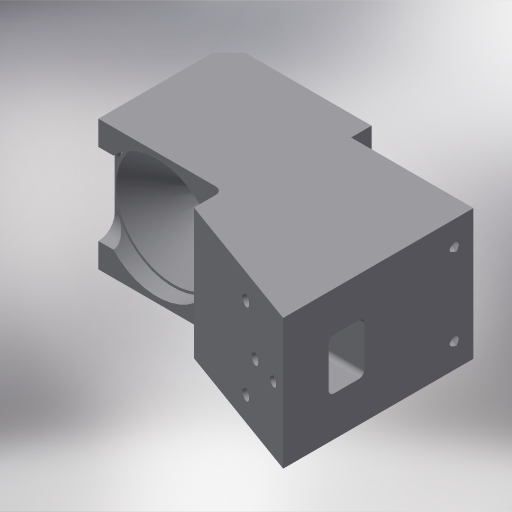
# Autodesk Inventor part: OdorBase_SideVacuumPort
Saved by Autodesk Inventor 2023 (Build 270158000, 158)
## iProperties
Created: 2008-10-04
Part Number: OdorBase_SideVacuumPort
Document SubType Name: Modeling
Designer: rinbergd
Density: 1 g/cm^3
Material: Generic
Appearance: Default
Author: osbornej
Autodesk Inventor part; units mm, degrees
ref_plane "YZ Plane" through (0, 0, 0) normal (1, 0, 0) x (0, 1, 0)
sketch "Sketch1" plane through (0, 0, 0) normal (0, 0, 1) x (1, 0, 0)
  line L0 (0, 24.892) -> (0, -24.892) projected
  line L1 (-25.6032, 0) -> (39.8272, 0) projected
  line L2 (30.48, -17.78) -> (-16.256, -17.78)
  line L3 (-16.256, -17.78) -> (-16.256, 17.78)
  line L4 (-16.256, 17.78) -> (30.48, 17.78)
  line L5 (30.48, 17.78) -> (30.48, -17.78)
  dimension "d0" = 30.48
  dimension "d1" = 16.256
  dimension "d2" = 17.78
  dimension "d3" = 35.56
  constraints: 8 end point, 2 parallel, 1 horizontal, 1 perpendicular
  measures "d0" distance between parallel lines of L5 L0
  measures "d1" distance between parallel lines of L3 L0
  measures "d2" distance between parallel lines of L1 L4
  measures "d3" distance of L2.end L3.end
extrude "Extrusion1" add sketch "Sketch1" along normal blind 45.72
sketch "Sketch2" plane through (-16.256, -17.78, 0) normal (0, -1, 0) x (1, 0, 0)
  line L0 (46.736, 45.72) -> (0, 45.72) projected
  line L1 (0, 0) -> (0, 45.72) projected
  line L2 (46.736, 0) -> (0, 0) projected
  line L3 (16.256, 54.864) -> (16.256, -9.144) projected
  line L4 (16.256, 45.72) -> (16.256, 20.32)
  line L5 (16.256, 20.32) -> (4.064, 20.32)
  line L6 (4.064, 20.32) -> (4.064, 23.368)
  arc A0 (4.064, 23.368) -> (0, 23.368) centre (2.032, 23.368) ccw
  line L7 (0, 23.368) -> (0, 45.72)
  line L8 (0, 45.72) -> (16.256, 45.72)
  line L9 (0, 2.54) -> (2.54, 0)
  line L10 (2.54, 0) -> (0, 0)
  line L11 (0, 0) -> (0, 2.54)
  dimension "d6" = 25.4
  dimension "d7" = 2.032
  dimension "d8" = 2.032
  dimension "d9" = 3.048
  dimension "d10" = 2.54
  dimension "d11" = 2.54
  dimension "d12" = 4.064
  constraints: 16 end point, 5 perpendicular, 5 point on line, 2 point on circle, 1 centre point, 1 collinear
  measures "d6" distance of L4.start L4.end
  measures "d7" radius of A0
  measures "d8" distance from line of L1 A0.centre
  measures "d9" distance from line of L5 A0.centre
  measures "d10" distance of L1.start L9.start
  measures "d11" distance of L9.end L1.start
  measures "d12" distance between parallel lines of L6 L7
extrude "Extrusion2" cut sketch "Sketch2" against normal through all contours L3 L5 L6 A0 L1 L0 | L9 L2 L1
sketch "Sketch3" plane through (-16.256, -17.78, 23.368) normal (-1, 0, 0) x (0, 0, 1)
  line L0 (-20.828, 35.56) -> (0, 35.56) projected
  line L1 (-20.828, 0) -> (0, 0) projected
  line L2 (-32.512, 17.78) -> (31.496, 17.78) projected
  line L3 (2.032, 35.56) -> (2.032, 0) projected
  line L4 (2.032, 35.56) -> (0, 35.56) projected
  line L5 (-23.368, 35.56) -> (-20.828, 35.56) projected
  line L6 (-20.828, 0) -> (-23.368, 0) projected
  line L7 (0, 0) -> (2.032, 0) projected
  line L8 (2.032, 0) -> (-23.368, 0)
  line L9 (-23.368, 0) -> (-23.368, 5.08)
  line L10 (-23.368, 5.08) -> (-3.048, 5.08)
  line L11 (-3.048, 5.08) -> (-3.048, 6.35)
  line L12 (-3.048, 6.35) -> (2.032, 6.35)
  line L13 (2.032, 6.35) -> (2.032, 0)
  line L14 (-20.828, 35.56) -> (0, 35.56)
  line L15 (-20.828, 35.56) -> (-23.368, 35.56)
  line L16 (0, 35.56) -> (2.032, 35.56)
  line L17 (2.032, 35.56) -> (-23.368, 35.56)
  line L18 (-23.368, 35.56) -> (-23.368, 30.48)
  line L19 (-23.368, 30.48) -> (-3.048, 30.48)
  line L20 (-3.048, 30.48) -> (-3.048, 29.21)
  line L21 (-3.048, 29.21) -> (2.032, 29.21)
  line L22 (2.032, 29.21) -> (2.032, 35.56)
  dimension "d15" = 6.35
  dimension "d16" = 5.08
  dimension "d17" = 5.08
  constraints: 30 end point, 4 perpendicular, 4 symmetric about line, 1 collinear, 1 parallel, 1 point on line
  measures "d15" distance of L12.end L3.end
  measures "d16" distance of L6.end L9.end
  measures "d17" distance between parallel lines of L11 L3
extrude "Extrusion3" cut sketch "Sketch3" against normal up to surface (16.256 mm away)
sketch "Sketch4" plane through (-16.256, -12.7, 2.54) normal (-1, 0, 0) x (0, 0, 1)
  line L0 (-11.684, 12.7) -> (52.324, 12.7) projected
  line L1 (22.86, 24.13) -> (22.86, 1.27) projected
  line L2 (22.86, 12.7) -> (22.86, 6.35)
  line L3 (17.78, 6.35) -> (22.86, 6.35)
  line L4 (15.24, 8.89) -> (15.24, 12.7)
  line L5 (15.24, 12.7) -> (22.86, 12.7)
  arc A0 (15.24, 8.89) -> (17.78, 6.35) centre (17.78, 8.89) ccw
  line L6 (22.86, 12.7) -> (22.86, 19.05)
  line L7 (17.78, 19.05) -> (22.86, 19.05)
  line L8 (15.24, 16.51) -> (15.24, 12.7)
  arc A1 (17.78, 19.05) -> (15.24, 16.51) centre (17.78, 16.51) ccw
  dimension "d20" = 2.54
  dimension "d21" = 6.35
  dimension "d22" = 7.62
  constraints: 14 end point, 4 point on circle, 4 symmetric about line, 3 perpendicular, 2 centre point, 2 point on line, 2 tangent, 1 midpoint, 1 other
  measures "d20" radius of A0
  measures "d21" distance of L2.start L2.end
  measures "d22" distance of L4.end L2.start
extrude "Extrusion4" cut sketch "Sketch4" against normal blind 7.874
sketch "Sketch11" plane through (0, -17.78, 0) normal (-1, 0, 0) x (0, 0, 1)
  line L0 (20.32, 5.08) -> (20.32, 30.48) projected
  line L1 (45.72, 35.56) -> (45.72, 0) projected
  line L2 (-9.144, 17.78) -> (54.864, 17.78) projected
  line L3 (20.32, 25.4) -> (20.32, 10.16) projected
  point P0 (20.32, 24.3791)
  point P1 (20.32, 11.1809)
  point P2 (43.18, 16.51)
  point P3 (43.18, 19.05)
  point P4 (23.368, 17.78)
  point P5 (22.733, 17.78)
  dimension "d73" = 1.27
  dimension "d74" = 1.27
  dimension "d75" = 2.54
  dimension "d76" = 2.54
  dimension "d78" = 0.635
  dimension "d476" = 2.413
  constraints: 2 point on line
  measures "d73" distance from line of point (43.18, 16.51) L2
  measures "d74" distance from line of point (43.18, 19.05) L2
  measures "d75" distance from line of point (43.18, 16.51) L1
  measures "d76" distance from line of point (43.18, 19.05) L1
  measures "d78" distance of point (22.733, 17.78) point (23.368, 17.78)
  measures "d476" distance from line of L0 point (22.733, 17.78)
hole "Hole3" at (0, 0, 22.733) direction (1, 0, 0) diameter 1.524 end through all
sketch "Sketch21" plane through (0, 0, 0) normal (0, 1, 0) x (-1, 0, 0)
  line L0 (0, -4.064) -> (0, 24.384) projected
  line L1 (13.716, 0) -> (0, 0) projected
  line L2 (16.256, 20.32) -> (16.256, 2.54) projected
  line L3 (4.3942, 0) -> (7.1374, 0)
  line L4 (4.3942, 0) -> (4.3942, 6.35)
  line L5 (4.3942, 6.35) -> (5.5499, 6.35)
  line L6 (5.5499, 6.35) -> (5.5499, 10.4775)
  line L7 (0, 20.32) -> (16.256, 20.32) projected
  line L8 (7.1374, 0) -> (7.1374, 20.32)
  line L9 (5.5499, 10.4775) -> (-1.7526, 17.78)
  line L10 (-1.7526, 17.78) -> (-1.7526, 20.32)
  line L11 (-1.7526, 20.32) -> (7.1374, 20.32)
  line L12 (-1.7526, 17.78) -> (-2.1495, 17.78)
  line L13 (-2.1495, 17.78) -> (-2.1495, 20.32)
  line L14 (-2.1495, 20.32) -> (-1.7526, 20.32)
  line L15 (-1.7526, 20.32) -> (-1.7526, 17.78)
  line L16 (5.5499, 8.4138) -> (7.1374, 8.4138)
  dimension "d159" = 7.1374
  dimension "d160" = 8.89
  dimension "d162" = 45
  dimension "d163" = 1.5875
  dimension "d292" = 0.3969
  dimension "d322" = 2.54
  constraints: 26 end point, 5 perpendicular, 5 point on line, 2 parallel, 1 collinear, 1 horizontal, 1 midpoint
  measures "d159" distance between parallel lines of L8 L0
  measures "d160" distance between parallel lines of L8 L10
  measures "d162" angle of L8 L9
  measures "d163" distance between parallel lines of L8 L6
  measures "d292" distance between parallel lines of L10 L13
  measures "d322" distance of L12.end L13.end
revolve "Revolution5" cut sketch "Sketch21" angle 360 about axis through (-7.1374, 0, 0) along (0, 0, 1) contours L9 L10 L11 L0 | L0 L7 L8 L16 L6 L9 | L4 L5 L6 L16 L8 L1 | L12 L13 L14 L10
sketch "Sketch23" plane through (0, 0, 0) normal (0, 0, -1) x (-1, 0, 0)
  line L0 (13.716, 12.7) -> (0, 12.7) projected
  line L1 (0, 17.78) -> (-30.48, 17.78) projected
  line L2 (-39.8272, 0) -> (25.6032, 0) projected
  line L3 (16.256, 12.7) -> (16.256, -12.7) projected
  line L4 (0, -12.7) -> (13.716, -12.7) projected
  line L5 (-30.48, -17.78) -> (0, -17.78) projected
  line L6 (8.382, -12.7) -> (8.382, -11.43)
  line L7 (-30.48, 17.78) -> (-30.48, -17.78) projected
  line L8 (8.382, -11.43) -> (-30.48, -11.43)
  line L9 (-30.48, -11.43) -> (-30.48, -17.78)
  line L10 (-30.48, -17.78) -> (8.382, -17.78)
  line L11 (8.382, -17.78) -> (8.382, -12.7)
  dimension "d193" = 7.874
  dimension "d231" = 6.35
  constraints: 10 end point, 3 perpendicular, 3 point on line
  measures "d193" distance between parallel lines of L3 L6
  measures "d231" distance between parallel lines of L8 L5
extrude "Extrusion12" cut sketch "Sketch23" against normal blind 27.94
mirror "Mirror5" about plane through (0, 0, 0) normal (0, 1, 0) of "Extrusion12"
sketch "Sketch32" plane through (0, 17.78, 45.72) normal (0, 1, 0) x (1, 0, 0)
  line L0 (30.48, 17.78) -> (0, 17.78) projected
  line L1 (0, 17.78) -> (0, 0) projected
  line L2 (0, 0) -> (30.48, 0) projected
  line L3 (30.48, 17.78) -> (30.48, 0) projected
extrude "Extrusion16" cut sketch "Sketch32" against normal up to surface (6.35 mm away)
sketch "Sketch33" plane through (0, -17.78, 45.72) normal (0, -1, 0) x (1, 0, 0)
  circle A0 centre (3.1266, -12.4245) radius 0.7366 projected
  line L0 (0, -17.78) -> (30.48, -17.78) projected
  line L1 (30.48, -17.78) -> (30.48, 0) projected
  line L2 (30.48, 0) -> (0, 0) projected
  line L3 (0, 0) -> (0, -17.78) projected
extrude "Extrusion17" cut sketch "Sketch33" against normal up to surface (6.35 mm away)
sketch "Sketch34" plane through (0, 11.43, 45.72) normal (0, 1, 0) x (1, 0, 0)
  line L0 (0, 0) -> (0, 25.4) projected
  line L1 (30.48, 0) -> (0, 0) projected
  line L2 (30.48, 45.72) -> (30.48, 0) projected
  line L3 (26.9647, 12.195) -> (4.5883, 20.3394) projected
  line L4 (26.9647, 12.195) -> (30.48, 10.9156)
  line L5 (4.5883, 20.3394) -> (0, 22.0094)
  point P0 (0, 24.13)
  constraints: 4 end point, 2 collinear, 2 point on line
extrude "Extrusion18" cut sketch "Sketch34" along normal through all both and the other way through all
sketch "Sketch35" plane through (-8.382, -11.43, 0) normal (0, -1, 0) x (1, 0, 0)
  line L0 (38.862, 34.8044) -> (8.382, 23.7106) projected
  line L1 (8.382, 20.32) -> (8.382, 23.7106) projected
  line L2 (38.862, 34.8044) -> (38.862, 0) projected
  line L3 (8.382, 20.32) -> (10.4457, 20.32)
  line L4 (11.557, 21.4312) -> (11.557, 24.8662)
  arc A0 (10.4457, 20.32) -> (11.557, 21.4312) centre (10.4457, 21.4312) ccw
  dimension "d284" = 1.1113
  dimension "d285" = 3.175
  constraints: 4 end point, 2 perpendicular, 2 point on circle, 2 point on line, 2 tangent, 1 centre point
  measures "d284" radius of A0
  measures "d285" distance between parallel lines of L4 L1
extrude "Extrusion19" cut sketch "Sketch35" against normal through all
sketch "Sketch38" plane through (0, 0, 0) normal (0, 0, -1) x (-1, 0, 0)
  line L0 (8.382, 11.43) -> (17.907, 11.43)
  line L1 (17.907, 11.43) -> (17.907, 14.605)
  line L2 (17.907, 14.605) -> (8.382, 14.605)
  line L3 (8.382, -11.43) -> (17.907, -11.43)
  line L4 (17.907, -11.43) -> (17.907, -14.605)
  line L5 (17.907, -14.605) -> (8.382, -14.605)
  line L6 (13.716, 12.7) -> (8.382, 12.7) projected
  line L7 (8.382, 11.43) -> (8.382, 14.605)
  line L8 (8.382, -11.43) -> (8.382, -14.605)
  dimension "d293" = 3.175
  dimension "d294" = 3.175
  dimension "d295" = 9.525
  constraints: 16 end point, 3 equal length, 3 perpendicular, 2 horizontal, 1 collinear
  measures "d293" distance of L0.end L1.end
  measures "d294" distance of L3.end L4.end
  measures "d295" distance of L1.end L2.end
extrude "Extrusion22" cut sketch "Sketch38" against normal through all
sketch "Sketch39" plane through (-16.256, -11.43, 2.54) normal (0, -1, 0) x (1, 0, 0)
  line L0 (4.064, 17.78) -> (18.3197, 17.78) projected
  line L1 (4.064, 20.828) -> (4.064, 17.78) projected
  arc A0 (4.064, 20.828) -> (0, 20.828) centre (2.032, 20.828) ccw projected
  line L2 (0, 0) -> (0, 20.828) projected
  line L3 (2.54, -2.54) -> (0, 0) projected
  line L4 (46.736, -2.54) -> (2.54, -2.54) projected
  line L5 (46.736, 32.2644) -> (46.736, -2.54) projected
  line L6 (46.736, 32.2644) -> (19.431, 22.3262) projected
  line L7 (19.431, 22.3262) -> (19.431, 18.8912) projected
  arc A1 (18.3197, 17.78) -> (19.431, 18.8912) centre (18.3197, 18.8912) ccw projected
  line L8 (4.4328, 17.78) -> (0, 17.78)
  constraints: 2 end point, 2 point on line, 1 perpendicular
extrude "Extrusion23" cut sketch "Sketch39" against normal through all contours L8 L2 A0 L1
sketch "Sketch45" plane through (-16.256, -11.43, 2.54) normal (0, -1, 0) x (1, 0, 0)
  line L0 (0, 17.78) -> (18.3197, 17.78) projected
  line L1 (0, 0) -> (0, 17.78) projected
  line L2 (2.54, -2.54) -> (0, 0) projected
  line L3 (46.736, -2.54) -> (2.54, -2.54) projected
  line L4 (46.736, 32.2644) -> (46.736, -2.54) projected
  line L5 (46.736, 32.2644) -> (19.431, 22.3262) projected
  line L6 (19.431, 22.3262) -> (19.431, 18.8912) projected
  arc A0 (18.3197, 17.78) -> (19.431, 18.8912) centre (18.3197, 18.8912) ccw projected
  circle A1 centre (2.3813, 7.62) radius 1.1906 projected
extrude "Extrusion29" cut sketch "Sketch45" against normal blind 1.27 contours L0 A0 L6 L5 L4 L3 L2 L1 | A1
sketch "Sketch46" plane through (-16.256, 11.43, 20.32) normal (0, 1, 0) x (1, 0, 0)
  line L0 (0, 0) -> (18.3197, 0) projected
  arc A0 (19.431, -1.1112) -> (18.3197, 0) centre (18.3197, -1.1112) ccw projected
  line L1 (19.431, -1.1112) -> (19.431, -4.5462) projected
  line L2 (19.431, -4.5462) -> (46.736, -14.4844) projected
  line L3 (46.736, 20.32) -> (46.736, -14.4844) projected
  line L4 (2.54, 20.32) -> (46.736, 20.32) projected
  line L5 (0, 17.78) -> (2.54, 20.32) projected
  line L6 (0, 0) -> (0, 17.78) projected
  circle A1 centre (2.3813, 10.16) radius 1.1906 projected
extrude "Extrusion30" cut sketch "Sketch46" against normal blind 1.27 contours L6 L5 L4 L3 L2 L1 A0 L0 | A1
sketch "Sketch47" plane through (-16.256, -10.16, 2.54) normal (0, -1, 0) x (1, 0, 0)
  line L0 (0, 0) -> (0, 17.78) projected
  line L1 (46.736, -2.54) -> (2.54, -2.54) projected
  line L2 (46.736, 32.2644) -> (46.736, -2.54) projected
  line L3 (19.431, 22.3262) -> (46.736, 32.2644) projected
  line L4 (0, 17.78) -> (18.3197, 17.78) projected
  line L5 (41.275, -2.54) -> (41.275, 30.2768)
  dimension "d327" = 41.275
  constraints: 2 end point, 2 point on line, 1 perpendicular
  measures "d327" distance between parallel lines of L5 L0
extrude "Extrusion31" cut sketch "Sketch47" against normal through all
sketch "Sketch49" plane through (0, 0, 0) normal (0, 0, -1) x (-1, 0, 0)
  circle A0 centre (-18.669, 0) radius 2.0574 projected
  line L0 (-5.969, -18.288) -> (-5.969, 13.462) projected
  line L1 (-31.369, -18.288) -> (-5.969, -18.288) projected
  line L2 (-31.369, -18.288) -> (-31.369, 13.462) projected
  line L3 (-31.369, 13.462) -> (-5.969, 13.462) projected
hole "Hole11" at (18.669, 0, 0) direction (0, 0, 1) diameter 3.6576 depth 7.9375 tip angle 118 clearance for "Flat Head Machine Screw (82)" size "#6" standard "Ansi Unified Screw Threads"
sketch "Sketch50" plane through (0, 0, 0) normal (0, 0, -1) x (-1, 0, 0)
  circle A0 centre (-18.669, 0) radius 1.8288 projected
  line L0 (13.716, 10.16) -> (-25.019, 10.16) projected
  line L1 (-25.019, 10.16) -> (-25.019, -10.16) projected
  line L2 (-25.019, -10.16) -> (13.716, -10.16) projected
  line L3 (-5.969, 10.16) -> (-5.969, -10.16)
  point P0 (-5.969, -10.16)
  point P1 (-5.969, 10.16)
  dimension "d340" = 19.05
  constraints: 2 end point, 2 point on line, 1 perpendicular
  measures "d340" distance between parallel lines of L3 L1
extrude "Extrusion33" cut sketch "Sketch50" against normal blind 3.175
sketch "Sketch51" plane through (25.019, -10.16, 32.8168) normal (1, 0, 0) x (0, 0, -1)
  circle A0 centre (10.0838, 10.16) radius 0.762 projected
  circle A1 centre (9.4488, 10.16) radius 0.508 projected
  line L0 (8.655, 8.5725) -> (11.0363, 8.5725)
  line L1 (11.0363, 8.5725) -> (11.0363, 11.7475)
  line L2 (11.0363, 11.7475) -> (8.655, 11.7475)
  line L3 (8.655, 11.7475) -> (8.655, 8.5725)
  circle A2 centre (8.655, 10.16) radius 1.5875
  circle A3 centre (11.0363, 10.16) radius 1.5875
  line L4 (-6.5634, 10.16) -> (39.3801, 10.16) projected
  line L5 (7.8613, 6.1913) -> (11.83, 6.1913)
  line L6 (12.6238, 6.985) -> (12.6238, 13.335)
  line L7 (11.83, 14.1288) -> (7.8613, 14.1288)
  line L8 (7.0675, 13.335) -> (7.0675, 6.985)
  arc A4 (7.0675, 7.7788) -> (8.655, 6.1913) centre (8.655, 7.7788) ccw
  arc A5 (12.6238, 13.335) -> (11.83, 14.1288) centre (11.83, 13.335) ccw
  arc A6 (11.83, 6.1913) -> (12.6238, 6.985) centre (11.83, 6.985) ccw
  arc A7 (7.8613, 14.1288) -> (7.0675, 13.335) centre (7.8613, 13.335) ccw
  arc A8 (7.0675, 6.985) -> (7.8613, 6.1913) centre (7.8613, 6.985) ccw
  dimension "d344" = 3.175
  dimension "d345" = 0
  dimension "d347" = 2.3813
  dimension "d352" = 0.9525
  dimension "d412" = 7.9375
  dimension "d413" = 3.9688
  dimension "d414" = 1.5875
  dimension "d415" = 0.7937
  constraints: 16 end point, 10 point on circle, 10 tangent, 5 centre point, 4 parallel, 3 equal radius, 2 horizontal, 2 midpoint, 2 perpendicular, 2 point on line, 2 vertical, 2 vertical alignment, 4 other
  measures "d344" distance between parallel lines of L2 L0
  measures "d345" distance from line of L4 point (11.036, 10.16)
  measures "d347" distance of L1.end L2.end
  measures "d352" distance from line of L1 A0.centre
  measures "d412" distance between parallel lines of L7 L5
  measures "d413" distance between parallel lines of L7 L4
  measures "d414" radius of A4
  measures "d415" radius of A5
extrude "Extrusion34" cut sketch "Sketch51" against normal blind 12.7
sketch "Sketch53" plane through (-16.256, -10.16, 2.54) normal (0, -1, 0) x (1, 0, 0)
  line L0 (0, 17.78) -> (18.3197, 17.78) projected
  line L1 (0, 17.78) -> (4.064, 17.78)
  line L2 (4.064, 17.78) -> (4.064, 20.828)
  line L3 (4.064, 20.828) -> (0, 20.828)
  line L4 (0, 20.828) -> (0, 17.78)
  circle A0 centre (2.032, 20.828) radius 2.032
  dimension "d353" = 4.064
  dimension "d354" = 3.048
  constraints: 8 end point, 2 parallel, 1 horizontal, 1 horizontal alignment, 1 midpoint, 1 perpendicular, 2 other
  measures "d353" distance of L2.end L3.end
  measures "d354" distance between parallel lines of L3 L0
extrude "Extrusion36" add sketch "Sketch53" against normal blind 3.81
sketch "Sketch54" plane through (-16.256, -10.16, 2.54) normal (0, -1, 0) x (1, 0, 0)
  line L0 (4.064, 17.78) -> (4.064, 20.828) projected
  arc A0 (4.064, 20.828) -> (0, 20.828) centre (2.032, 20.828) ccw projected
  line L1 (0, 20.828) -> (0, 0) projected
  line L2 (2.54, -2.54) -> (0, 0) projected
  line L3 (22.225, -2.54) -> (2.54, -2.54) projected
  line L4 (4.064, 17.78) -> (4.064, -2.54)
  constraints: 2 end point, 1 perpendicular, 1 point on line
extrude "Extrusion37" add sketch "Sketch54" along normal blind 3.175
sketch "Sketch55" plane through (-16.256, -13.335, 2.54) normal (0, -1, 0) x (1, 0, 0)
  arc A0 (4.064, 20.828) -> (0, 20.828) centre (2.032, 20.828) ccw projected
  point P0 (2.032, 20.828)
  constraints: 1 coincident
hole "Hole12" at (-14.224, -13.335, 23.368) direction (0, 1, 0) diameter 1.1906 depth 9.525 counterbore diameter 3.048 counterbore depth 5.334
sketch "Sketch56" plane through (2.0637, 1.2589, 20.32) normal (0, 0, 1) x (1, 0, 0)
  arc A0 (0, 0) -> (0, -2.5178) centre (-9.2011, -1.2589) ccw projected
  circle A1 centre (-9.2011, -1.2589) radius 9.2869
  point P0 (-14.2557, 6.5319)
  constraints: 1 centre point, 1 coincident, 1 concentric
extrude "Extrusion38" cut sketch "Sketch56" along normal blind 25.4
sketch "Sketch60" plane through (-16.256, -13.335, 2.54) normal (0, -1, 0) x (1, 0, 0)
  circle A0 centre (2.032, 20.828) radius 1.524 projected
  line L0 (4.064, 20.828) -> (4.064, -2.54) projected
  arc A1 (4.064, 20.828) -> (0, 20.828) centre (2.032, 20.828) ccw projected
  line L1 (0, 0) -> (0, 20.828) projected
  line L2 (0, 17.653) -> (4.064, 17.653)
  dimension "d378" = 3.175
  constraints: 2 end point, 2 point on line, 1 perpendicular
  measures "d378" distance from line of A0.centre L2
extrude "Extrusion41" cut sketch "Sketch60" against normal blind 1.27
sketch "Sketch62" plane through (-16.256, -13.335, 2.54) normal (0, -1, 0) x (1, 0, 0)
  line L0 (4.064, 11.303) -> (0, 11.303) projected
  line L1 (0, 0) -> (0, 17.653) projected
  line L2 (2.54, -2.54) -> (0, 0) projected
  line L3 (4.064, -2.54) -> (2.54, -2.54) projected
  line L4 (4.064, 17.653) -> (4.064, -2.54) projected
extrude "Extrusion43" cut sketch "Sketch62" against normal up to surface (3.175 mm away)
fillet "Fillet2" radius 0.4001 1 edges at (-14.224, -12.065, 20.193)
ref_plane "Work Plane10" through (-16.256, -14.605, 2.54) normal (0, -1, 0) x (1, 0, 0)
sketch "Sketch63" plane through (-16.256, -14.605, 2.54) normal (0, -1, 0) x (1, 0, 0)
  line L0 (0, 17.653) -> (4.064, 17.653) projected
  line L1 (0, 11.303) -> (0, 17.653) projected
  point P0 (2.032, 14.478)
  dimension "d387" = 3.175
  dimension "d388" = 2.032
  measures "d387" distance from line of point (2.032, 14.478) L0
  measures "d388" distance from line of point (2.032, 14.478) L1
hole "Hole13" at (-14.224, -14.605, 17.018) direction (0, 1, 0) diameter 2.159 depth 3.175 tip angle 118
mirror "Mirror8" about plane through (0, 0, 0) normal (0, 1, 0) of "Hole12", "Extrusion38", "Extrusion37", "Extrusion36", "Extrusion41", "Extrusion43", "Fillet2", "Hole13"
pattern_linear "Rectangular Pattern1" count 2 spacing 2.54 along (0, 1, 0) of "Hole3"
pattern_linear "Rectangular Pattern2" count 2 spacing 2.54 along (0, -1, 0) of "Hole3"
sketch "Sketch65" plane through (-16.256, -3.81, 17.78) normal (-1, 0, 0) x (0, 0, 1)
  line L0 (-3.937, 13.97) -> (8.3591, 13.97)
  line L1 (8.3591, 13.97) -> (8.3591, 19.1782)
  line L2 (8.3591, 19.1782) -> (-3.937, 19.1782)
  line L3 (-3.937, 19.1782) -> (-3.937, 13.97)
  line L4 (-4.3371, -6.35) -> (8.3591, -6.35)
  line L5 (8.3591, -6.35) -> (8.3591, -11.3681)
  line L6 (8.3591, -11.3681) -> (-4.3371, -11.3681)
  line L7 (-4.3371, -11.3681) -> (-4.3371, -6.35)
  line L8 (8.3591, 19.1782) -> (2.54, 19.1782)
  line L9 (2.54, 19.1782) -> (2.54, 10.16)
  line L10 (2.54, 10.16) -> (8.3591, 10.16)
  line L11 (8.3591, 10.16) -> (8.3591, 19.1782)
  line L12 (8.3591, -11.3681) -> (2.54, -11.3681)
  line L13 (2.54, -11.3681) -> (2.54, -2.54)
  line L14 (2.54, -2.54) -> (8.3591, -2.54)
  line L15 (8.3591, -2.54) -> (8.3591, -11.3681)
  constraints: 32 end point, 8 parallel, 4 horizontal, 4 perpendicular, 1 collinear
extrude "Extrusion44" cut sketch "Sketch65" against normal up to surface (4.064 mm away)
ref_plane "Work Plane6" through (-7.1374, 0, 10.4775) normal (0, -1, 0) x (0, 0, -1)
sketch "Sketch68" plane through (-16.256, -3.81, 17.78) normal (0, 0, 1) x (1, 0, 0)
  line L0 (0, 7.62) -> (0.6492, 7.62) projected
  line L1 (0, 0) -> (0, 7.62) projected
  line L2 (0, 0) -> (0.6492, 0) projected
  arc A0 (0.6492, 0) -> (0.6492, 7.62) centre (9.1186, 3.81) ccw projected
extrude "Extrusion47" cut sketch "Sketch68" along normal blind 25.4
sketch "Sketch71" plane through (3.175, -10.16, 24.8662) normal (-0.3420201, 0, 0.9396926) x (0.9396926, 0, 0.3420201)
  circle A0 centre (13.4938, 16.51) radius 1.2192
  circle A1 centre (13.4938, 3.81) radius 1.2192
  point P0 (-11.4883, 10.16)
  constraints: 2 centre point, 2 coincident, 4 other
hole "Hole14" at (15.855, -6.35, 29.4814) at (15.855, 6.35, 29.4814) direction (0.3420201, 0, -0.9396926) diameter 1.778 depth 25.4 tip angle 118 clearance for "Flat Head Machine Screw (82)" size "#0" standard "Ansi Unified Screw Threads"
sketch "Sketch77" plane through (3.175, -10.16, 24.8662) normal (-0.3420201, 0, 0.9396926) x (0.9396926, 0, 0.3420201)
  line L0 (33.2479, 10.16) -> (-36.7659, 10.16) projected
  line L1 (23.2459, 0) -> (23.2459, 20.32) projected
  point P0 (-11.4883, 10.16)
  point P1 (20.6297, 10.16)
  dimension "d460" = 2.6162
  constraints: 1 point on line
  measures "d460" distance from line of point (20.63, 10.16) L1
hole "Hole15" at (22.5606, 0, 31.922) direction (0.3420201, 0, -0.9396926) diameter 1.5875 depth 3.175 tip angle 118
sketch "Sketch78" plane through (3.175, -10.16, 24.8662) normal (-0.3420201, 0, 0.9396926) x (0.9396926, 0, 0.3420201)
  line L0 (33.2479, 10.16) -> (-36.7659, 10.16) projected
  line L1 (23.2459, 0) -> (23.2459, 20.32) projected
  point P0 (-11.4883, 10.16)
  point P1 (15.8799, 10.16)
  dimension "d468" = 7.366
  constraints: 1 point on line
  measures "d468" distance from line of point (15.88, 10.16) L1
hole "Hole16" at (18.0972, 0, 30.2975) direction (0.3420201, 0, -0.9396926) diameter 1.778 depth 2.3813 tip angle 118 clearance for "Flat Head Machine Screw (82)" size "#0" standard "Ansi Unified Screw Threads"
sketch "Sketch80" plane through (0, 0, 0) normal (0, 0, -1) x (-1, 0, 0)
  circle A0 centre (7.1374, 0) radius 2.9281
  point P0 (0, 0)
  constraints: 1 centre point, 1 coincident
extrude "Extrusion50" add sketch "Sketch80" against normal blind 6.35
sketch "Sketch81" plane through (-16.256, -10.16, 2.54) normal (0, -1, 0) x (1, 0, 0)
  line L0 (0, 17.78) -> (18.3197, 17.78) projected
  line L1 (0, 0) -> (0, 17.78) projected
  point P0 (16.256, -2.54)
  point P1 (9.525, 5.08)
  dimension "d486" = 12.7
  dimension "d487" = 9.525
  measures "d486" distance from line of point (9.525, 5.08) L0
  measures "d487" distance from line of L1 point (9.525, 5.08)
hole "Hole17" at (-6.731, -10.16, 7.62) direction (0, 1, 0) diameter 5.3594 depth 12.7 tip angle 118 thread size "1/4-28 UNF" class "2B" standard "ANSI Unified Screw Threads"
equation "\"d2\" = 0.5 * d3"
body "Solid1"
